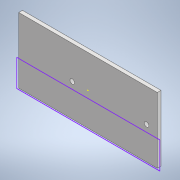
# Autodesk Inventor part: rails stock solid
Saved by Autodesk Inventor 2020 (Build 240168000, 168)
## iProperties
Created: 2019-05-20
Part Number: rails stock solid
Material: Generic
Document SubType Name: Modeling
Designer: LillaHunden
Density: 1 g/cm^3
Appearance: Default
Author: LillaHunden
Autodesk Inventor part; units mm, degrees
ref_plane "YZ Plane" through (0, 0, 0) normal (1, 0, 0) x (0, 1, 0)
ref_plane "XZ Plane" through (0, 0, 0) normal (0, 1, 0) x (-1, 0, 0)
ref_plane "XY Plane" through (0, 0, 0) normal (0, 0, 1) x (1, 0, 0)
sketch "Sketch1" plane through (0, 0, 0) normal (0, 0, 1) x (1, 0, 0)
  point P0 (0, 0)
sketch "Sketch2" plane through (0, 0, 0) normal (0, 0, 1) x (1, 0, 0)
  line L0 (-186, -88) -> (186, -88)
  line L1 (186, -88) -> (186, 88)
  line L2 (186, 88) -> (-186, 88)
  line L3 (-186, 88) -> (-186, -88)
  line L4 (-186, -88) -> (186, 88) construction
  line L5 (186, -88) -> (-186, 88) construction
  point P0 (0, 0)
  dimension "d0" = 372
  dimension "d1" = 176
  constraints: 12 end point, 2 midpoint, 2 parallel, 1 horizontal, 1 perpendicular
  measures "d0" distance of L2.end L1.end
  measures "d1" distance of L1.end L0.end
extrude "Extrusion1" add sketch "Sketch2" along normal blind 10
sketch "Sketch3" plane through (0, 0, 10) normal (0, 0, 1) x (1, 0, 0)
  circle A0 centre (157.07, -0.5) radius 6
  circle A1 centre (-42.47, -0.5) radius 6
  line L0 (163.07, 41.41) -> (163.07, 2.6213) construction
  line L1 (-36.47, 12.5914) -> (-36.47, -19.2897) construction
  line L2 (186, -88) -> (186, 88) construction
  line L3 (-48.47, 40.0816) -> (-48.47, 5.69) construction
  line L4 (-186, 88) -> (-186, -88) construction
  line L5 (145.9116, -6.5) -> (169.2139, -6.5) construction
  line L6 (-62.3973, -6.5) -> (-31.6806, -6.5) construction
  line L7 (-186, -88) -> (186, -88) construction
  point P0 (0, 0)
  dimension "d4" = 12
  dimension "d5" = 12
  dimension "d6" = 22.93
  dimension "d7" = 137.53
  dimension "d8" = 81.5
  constraints: 10 end point, 5 tangent, 3 vertical, 2 centre point, 1 horizontal, 1 horizontal alignment, 1 perpendicular
  measures "d4" diameter of A0
  measures "d5" diameter of A1
  measures "d6" distance between parallel lines of L2 L0
  measures "d7" distance between parallel lines of L4 L3
  measures "d8" distance between parallel lines of L7 L5
extrude "Extrusion2" cut sketch "Sketch3" against normal through all
sketch "Sketch4" plane through (0, 0, 10) normal (0, 0, 1) x (1, 0, 0)
  line L0 (-107.2483, -51.5859) -> (189.4561, -51.5859)
  line L1 (189.4561, -51.5859) -> (189.4561, -65.196)
  line L2 (189.4561, -65.196) -> (-107.2483, -65.196)
  line L3 (-107.2483, -65.196) -> (-107.2483, -51.5859)
  point P0 (0, 0)
  constraints: 8 end point, 2 parallel, 1 horizontal, 1 perpendicular
body "Solid1"
